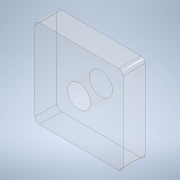
# Autodesk Inventor part: 104.001.01_Auflageplatte_FB
Saved by Autodesk Inventor 2021 (Build 250183000, 183)
## iProperties
Created: 2021-11-27
Part Number: 104.001.01_Auflageplatte_FB
Material: PMMA-Kunststoff
Document SubType Name: Modeling
Designer: Sebastian Seewald
Mass: 2.24475 g
Surface Area: 12.2891 cm^2
Volume: 1.88952 cm^3
Density: 1.188 g/cm^3
Appearance: Polycarbonat - klar
Author: Sebastian Seewald
Autodesk Inventor part; units mm, degrees
ref_plane "YZ Plane" through (0, 0, 0) normal (1, 0, 0) x (0, 1, 0)
ref_plane "XZ Plane" through (0, 0, 0) normal (0, 1, 0) x (-1, 0, 0)
ref_plane "XY Plane" through (0, 0, 0) normal (0, 0, 1) x (1, 0, 0)
sketch "Skizze1" plane through (0, 0, 0) normal (0, 0, 1) x (1, 0, 0)
  line L0 (1, 0) -> (19, 0)
  line L1 (20, 1) -> (20, 19)
  line L2 (19, 20) -> (1, 20)
  line L3 (0, 19) -> (0, 1)
  arc A0 (1, 20) -> (0, 19) centre (1, 19) ccw
  arc A1 (0, 1) -> (1, 0) centre (1, 1) ccw
  arc A2 (19, 0) -> (20, 1) centre (19, 1) ccw
  arc A3 (20, 19) -> (19, 20) centre (19, 19) ccw
  circle A4 centre (10, 10) radius 2.6
  point P0 (0, 0)
  point P1 (20, 20)
  point P2 (20, 0)
  point P3 (0, 20)
  dimension "d0" = 20
  dimension "d1" = 20
  dimension "d2" = 1
  dimension "d3" = 5.2
  dimension "d4" = 10
  dimension "d5" = 10
  constraints: 8 end point, 8 point on circle, 8 point on line, 8 tangent, 5 centre point, 3 equal radius, 2 parallel, 1 horizontal, 1 perpendicular
  measures "d0" distance of point (20, 20) point (0, 20)
  measures "d1" distance of point (20, 0) point (20, 20)
  measures "d2" radius of A0
  measures "d3" diameter of A4
  measures "d4" distance from line of L3 A4.centre
  measures "d5" distance from line of L0 A4.centre
extrude "Extrusion1" add sketch "Skizze1" along normal blind 5
